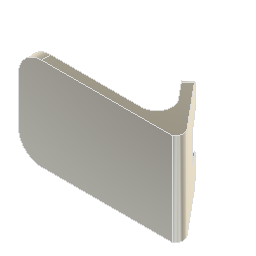
Держатель ложки-вилки на кухню (Autodesk Fusion 360 design; units mm, degrees)
Autodesk Fusion 360 part; units mm, degrees
sketch "Sketch1" plane through (0, 0, 0) normal (0, 0, 1) x (1, 0, 0)
  line L0 (0, 0) -> (36.8248, 0)
  line L1 (50, -3) -> (0, -3)
  line L2 (0, -3) -> (0, 0)
  line L3 (40.6659, 8.2009) -> (35, 15)
  line L4 (50.3841, 1.2252) -> (37.3047, 16.9206)
  line L5 (35, 15) -> (37.3047, 16.9206)
  arc A0 (50, -3) -> (50.3841, 1.2252) centre (48.0794, -0.6953) ccw
  arc A1 (36.8248, 0) -> (40.6659, 8.2009) centre (36.8248, 5) ccw
  dimension "d1" = 3
  dimension "d3" = 3
  dimension "d4" = 5
  constraint horizontal L0
  constraint horizontal L1
  constraint vertical L2
  constraint coincident L0.start L2.end
  constraint perpendicular L4 L5
  constraint tangent L4 A0
  constraint coincident L1.start A0.start
  constraint tangent L3 A1
  constraint tangent L0 A1
  measures "d1" distance of L0.start L1.end
  measures "d3" radius of A0
  measures "d4" radius of A1
extrude "Extrude1" add sketch "Sketch1" along normal blind 30
sketch "Sketch2" plane through (0, 0, 0) normal (1, 0, 0) x (0, 1, 0)
  line L0 (0, 0) -> (0, 30)
  line L1 (0, 10) -> (25, 10)
  line L2 (0, 20) -> (25, 20)
  line L3 (11, 10) -> (11, 20)
  line L4 (20, 10) -> (20, 20)
  constraint coincident L0.start origin
  constraint vertical L0
  constraint coincident L1 L3.start
  constraint coincident L2 L3.end
  constraint perpendicular L2 L3
  constraint coincident L1 L4.start
  constraint coincident L2 L4.end
  constraint perpendicular L2 L4
extrude "Extrude2" cut sketch "Sketch2" along normal blind 58 contours L1 L2 L3 L4
fillet "Fillet1" radius 1.5 2 edges at (36.1523, 15.9603, 20) (36.1523, 15.9603, 10)
fillet "Fillet2" radius 1.5 2 edges at (40.2859, 11, 20) (40.2859, 11, 10)
fillet "Fillet3" radius 2 2 edges at (36.1523, 15.9603, 0) (36.1523, 15.9603, 30)
fillet "Fillet4" radius 7.5 2 edges at (0, -1.5, 0) (0, -1.5, 30)
